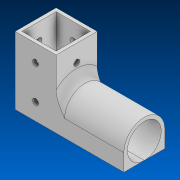
# Autodesk Inventor part: Tracking Wheel Guide
Saved by Autodesk Inventor 2022.2 (Build 262287000, 287)
## iProperties
Created: 2022-03-25
Part Number: Tracking Wheel Guide
Material: Generic
Document SubType Name: Modeling
Designer: omard
Density: 1 g/cm^3
Appearance: Default
Author: omard
Autodesk Inventor part; units mm, degrees
ref_plane "YZ Plane" through (0, 0, 0) normal (1, 0, 0) x (0, 1, 0)
ref_plane "XZ Plane" through (0, 0, 0) normal (0, 1, 0) x (-1, 0, 0)
ref_plane "XY Plane" through (0, 0, 0) normal (0, 0, 1) x (1, 0, 0)
sketch "Sketch1" plane through (0, 0, 0) normal (0, 1, 0) x (-1, 0, 0)
  line L0 (12.827, 12.827) -> (-12.827, 12.827)
  line L1 (-12.827, 12.827) -> (-12.827, -12.827)
  line L2 (-12.827, -12.827) -> (12.827, -12.827)
  line L3 (12.827, -12.827) -> (12.827, 12.827)
  line L4 (12.827, 12.827) -> (-12.827, -12.827) construction
  line L5 (-12.827, 12.827) -> (12.827, -12.827) construction
  line L6 (15.367, 15.367) -> (-15.367, 15.367)
  line L7 (-15.367, 15.367) -> (-15.367, -15.367)
  line L8 (-15.367, -15.367) -> (15.367, -15.367)
  line L9 (15.367, -15.367) -> (15.367, 15.367)
  point P0 (0, 0)
  dimension "d0" = 25.654
  dimension "d1" = 25.654
  dimension "d2" = 2.54
  constraints: 20 end point, 4 parallel, 2 midpoint, 2 perpendicular, 1 horizontal, 3 other
  measures "d0" distance of L2.end L1.end
  measures "d1" distance of L1.end L0.end
  measures "d2" distance between parallel lines of L3 L9
extrude "Extrusion1" add sketch "Sketch1" along normal blind 50.8
sketch "Sketch2" plane through (15.367, 0, 15.367) normal (1, 0, 0) x (0, 0, -1)
  line L0 (0, 50.8) -> (30.734, 50.8) projected
  point P0 (15.367, 0)
  point P1 (15.367, 12.7)
  point P2 (15.367, 38.1)
  point P3 (15.367, 50.8)
  dimension "d5" = 12.7
  dimension "d6" = 25.4
  constraints: 2 vertical alignment, 1 midpoint
  measures "d5" distance from line of L0 point (15.367, 38.1)
  measures "d6" distance of point (15.367, 38.1) point (15.367, 12.7)
hole "Hole1" at (15.367, 12.7, 0) at (15.367, 38.1, 0) direction (-1, 0, 0) diameter 4.445 end through all start extended yes
sketch "Sketch3" plane through (-15.367, 0, 15.367) normal (0, 0, 1) x (1, 0, 0)
  line L0 (0, 50.8) -> (30.734, 50.8) projected
  point P0 (15.367, 0)
  point P1 (15.367, 12.7)
  point P2 (15.367, 38.1)
  point P3 (30.734, 38.1)
  point P4 (30.734, 12.7)
  point P5 (15.367, 50.8)
  constraints: 2 horizontal alignment, 2 vertical alignment, 1 midpoint
hole "Hole2" at (0, 38.1, 15.367) at (0, 12.7, 15.367) direction (0, 0, -1) diameter 4.445 end through all start extended yes
sketch "Sketch4" plane through (15.367, 0, 15.367) normal (1, 0, 0) x (0, 0, -1)
  circle A0 centre (15.367, 12.7) radius 2.2225 projected
  circle A1 centre (15.367, 12.7) radius 12.7
  circle A2 centre (15.367, 12.7) radius 15.367
  line L0 (30.734, 0) -> (30.734, 50.8) projected
  line L1 (0, 0) -> (30.734, 0) projected
  line L2 (0, 0) -> (0, 50.8) projected
  point P0 (15.367, 0)
  point P1 (0, 12.7)
  point P2 (30.734, 12.7)
  constraints: 2 coincident, 1 centre point, 1 tangent, 1 vertical alignment, 2 other
extrude "Extrusion2" add sketch "Sketch4" along normal blind 50.8 contours L1 A2 | L1 L2 A2 | A2 L0 L1 picked at (29.6962, 13.9259)
extrude "Extrusion3" cut sketch "Sketch4" against normal up to surface (28.194 mm away) contours A1
fillet "Fillet1" radius 6.35 1 edges at (15.367, 28.067, 0)
body "Solid1"
